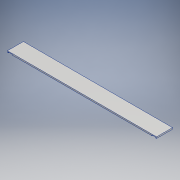
# Autodesk Inventor part: 앞판_위
Saved by Autodesk Inventor 2017 (Build 210142000, 142)
## iProperties
Part Number: 앞판_위
Material: 알루미늄 6061
Document SubType Name: Modeling
Designer: minom
Density: 2.7 g/cm^3
Appearance: 알루미늄 - 평지
Mass: 23.8313 g
Surface Area: 100.424 cm^2
Volume: 8.8264 cm^3
Author: minom
Autodesk Inventor part; units mm, degrees
ref_plane "YZ Plane" through (0, 0, 0) normal (1, 0, 0) x (0, 1, 0)
ref_plane "XZ Plane" through (0, 0, 0) normal (0, 1, 0) x (-1, 0, 0)
ref_plane "XY Plane" through (0, 0, 0) normal (0, 0, 1) x (1, 0, 0)
sketch "스케치1" plane through (0, 0, 0) normal (0, 0, 1) x (1, 0, 0)
  line L0 (-190, 35) -> (16, 35)
  line L1 (16, 35) -> (16, 13)
  line L2 (16, 13) -> (-190, 13)
  line L3 (-190, 13) -> (-190, 35)
  point P0 (0, 0)
  dimension "d0" = 206
  dimension "d1" = 22
  constraints: 8 end point, 2 parallel, 1 horizontal, 1 perpendicular
  measures "d0" distance of L1.end L2.end
  measures "d1" distance of L0.end L1.end
extrude "돌출1" add sketch "스케치1" along normal blind 2
sketch "스케치2" plane through (0, 0, 0) normal (0, 0, -1) x (-1, 0, 0)
  line L0 (-16, 35) -> (190, 35) projected
  line L1 (190, 13) -> (-16, 13) projected
  line L2 (-15, 35) -> (-9.6, 35)
  line L3 (-9.6, 35) -> (-9.6, 13)
  line L4 (-9.6, 13) -> (-15, 13)
  line L5 (-15, 13) -> (-15, 35)
  line L6 (189, 35) -> (183.6, 35)
  line L7 (183.6, 35) -> (183.6, 13)
  line L8 (183.6, 13) -> (189, 13)
  line L9 (189, 13) -> (189, 35)
  line L10 (190, 13) -> (190, 35) projected
  line L11 (-16, 35) -> (-16, 13) projected
  point P0 (0, 0)
  dimension "d4" = 5.4
  dimension "d5" = 5.4
  dimension "d6" = 1
  dimension "d7" = 1
  constraints: 16 end point, 4 parallel, 4 point on line, 2 horizontal, 2 perpendicular
  measures "d4" distance of L3.end L4.end
  measures "d5" distance of L8.end L7.end
  measures "d6" distance between parallel lines of L9 L10
  measures "d7" distance between parallel lines of L5 L11
extrude "돌출2" cut sketch "스케치2" against normal blind 1 contours L0 L3 L1 L5 | L0 L9 L1 L7
